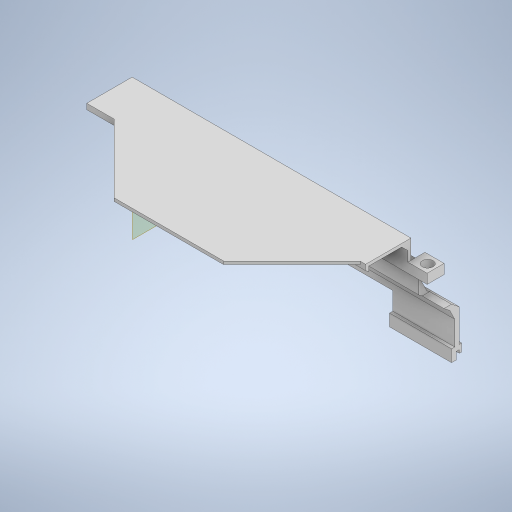
# Autodesk Inventor part: kryt
Saved by Autodesk Inventor 2024 (Build 280153000, 153)
## iProperties
Created: 2023-09-06
Part Number: kryt
Material: Všeobecné
Document SubType Name: Modeling
Designer: Simak
Density: 1 g/cm^3
Appearance: Výchozí
Author: Simak
Autodesk Inventor part; units mm, degrees
ref_plane "YZ Plane" through (0, 0, 0) normal (1, 0, 0) x (0, 1, 0)
ref_plane "XZ Plane" through (0, 0, 0) normal (0, 1, 0) x (-1, 0, 0)
ref_plane "XY Plane" through (0, 0, 0) normal (0, 0, 1) x (1, 0, 0)
ref_plane "Pracovní rovina12" through (0, 3, 0) normal (0, 1, 0) x (1, 0, 0)
sketch "Náčrt28" plane through (0, 3, 0) normal (0, 1, 0) x (1, 0, 0)
  circle A0 centre (-42.25, 8.5) radius 1.85
  circle A1 centre (42.25, 8.5) radius 1.85
  circle A2 centre (42.25, -29) radius 1.85
  circle A3 centre (-42.25, -29) radius 1.85
  line L0 (-42.25, 8.5) -> (-49.75, 8.5) construction
  line L1 (-49.75, 19.25) -> (-49.75, -49.75) projected
  line L2 (42.25, 8.5) -> (49.75, 8.5) construction
  line L3 (49.75, -49.75) -> (49.75, 19.25) projected
  line L4 (-49.75, -49.75) -> (49.75, -49.75) projected
  point P0 (0, 0)
  dimension "d185" = 3.7
  dimension "d186" = 84.5
  dimension "d187" = 37.5
  dimension "d195" = 20.75
  constraints: 4 centre point, 4 end point, 3 equal radius, 3 point on line, 2 horizontal alignment, 2 vertical alignment, 1 collinear, 1 horizontal
  measures "d185" diameter of A0
  measures "d186" distance of L2.start L0.start
  measures "d187" distance of A3.centre L0.start
  measures "d195" distance from line of L4 A3.centre
ref_plane "Pracovní rovina6" through (49.75, 0, 49.75) normal (1, 0, 0) x (0, 0, -1)
sketch "Náčrt29" plane through (49.75, 0, 49.75) normal (1, 0, 0) x (0, 0, -1)
  line L0 (0, 0) -> (69, 0) projected
  line L1 (0, 0) -> (6.6987, 25)
  line L2 (6.6987, 25) -> (9.8046, 25)
  line L3 (9.8046, 25) -> (3.9097, 3)
  line L4 (0, 3) -> (69, 3) projected
  line L5 (0, 0) -> (0, 3) projected
  point P0 (49.75, 0)
  point P1 (0.8038, 3)
  dimension "d188" = 75
  dimension "d189" = 25
  dimension "d190" = 3
  constraints: 6 end point, 1 horizontal, 1 parallel, 1 point on line
  measures "d188" angle of L0 L1
  measures "d189" distance between parallel lines of L0 L2
  measures "d190" distance between parallel lines of L1 L3
ref_plane "Pracovní rovina7" through (-49.75, 25, 5) normal (0, 0, 1) x (1, 0, 0)
sketch "Náčrt49" plane through (-49.75, 25, 5) normal (0, 0, 1) x (1, 0, 0)
  line L0 (0, 0) -> (2.5, 0) projected
  line L1 (1.25, 0) -> (4.45, 0)
  line L2 (4.45, 0) -> (4.45, 5.2)
  line L3 (4.45, 5.2) -> (1.25, 5.2)
  line L4 (1.25, 5.2) -> (1.25, 0)
  line L5 (2.5, 7.2) -> (6.45, 7.2)
  line L6 (6.45, 7.2) -> (6.45, -2)
  line L7 (6.45, -2) -> (2.5, -2)
  line L8 (2.5, 7.2) -> (2.5, 5.2)
  line L9 (2.5, 0) -> (2.5, -12) projected
  line L10 (2.5, 0) -> (2.5, -2)
  line L11 (2.5, 0) -> (2.5, 19) projected
  point P0 (49.75, -25)
  point P1 (1.25, 0)
  point P2 (2.5, 0)
  point P3 (2.5, 0)
  dimension "d289" = 3.2
  dimension "d290" = 5.2
  dimension "d291" = 2
  dimension "d292" = 2
  dimension "d293" = 2
  constraints: 18 end point, 3 perpendicular, 2 collinear, 2 horizontal, 2 midpoint, 2 parallel, 1 point on line, 1 vertical, 1 vertical alignment
  measures "d289" distance of L2.end L3.end
  measures "d290" distance of L1.end L2.end
  measures "d291" distance between parallel lines of L1 L7
  measures "d292" distance between parallel lines of L6 L2
  measures "d293" distance between parallel lines of L3 L5
ref_plane "Pracovní rovina14" through (0, 0, 0) normal (0, -1, 0) x (1, 0, 0)
sketch "Náčrt53" plane through (0, 0, 0) normal (0, -1, 0) x (1, 0, 0)
  line L0 (5, -49.75) -> (-5, -49.75) projected
  line L1 (-5, -49.75) -> (-5, -39.875) projected
  line L2 (-5, -39.875) -> (5, -39.875) projected
  line L3 (5, -39.875) -> (5, -49.75) projected
  line L4 (0, -48.0745) -> (-2.825, -46.4435)
  line L5 (-2.825, -46.4435) -> (-2.825, -43.1815)
  line L6 (-2.825, -43.1815) -> (0, -41.5505)
  line L7 (0, -41.5505) -> (2.825, -43.1815)
  line L8 (2.825, -43.1815) -> (2.825, -46.4435)
  line L9 (2.825, -46.4435) -> (0, -48.0745)
  line L10 (0, -48.0745) -> (0, -49.75) construction
  line L11 (0, -41.5505) -> (0, -39.875) construction
  circle A0 centre (0, -44.8125) radius 1.85
  point P0 (0, 0)
  point P1 (0, -44.8125)
  dimension "d328" = 3.7
  dimension "d389" = 5.65
  constraints: 16 end point, 2 midpoint, 1 centre point, 1 coincident, 1 collinear, 1 vertical, 1 vertical alignment, 13 other
  measures "d328" diameter of A0
  measures "d389" distance between parallel lines of L8 L5
ref_plane "Pracovní rovina10" through (27, 7.646, -39.875) normal (1, 0, 0) x (0, 0, -1)
sketch "Náčrt72" plane through (27, 7.646, -39.875) normal (1, 0, 0) x (0, 0, -1)
  line L0 (-1.9585, -1.746) -> (-8.7915, -1.746)
  line L1 (-8.7915, 8.454) -> (-1.9585, 8.454)
  arc A0 (-8.7915, 8.454) -> (-8.7915, -1.746) centre (-5.375, 3.354) ccw
  arc A1 (-1.9585, -1.746) -> (-1.9585, 8.454) centre (-5.375, 3.354) ccw
  line L2 (-9, -7.646) -> (-1, -7.646) projected
  line L3 (-10.75, 0) -> (-10.75, 3.354) projected
  arc A2 (-10.75, 0) -> (-5.375, -3.1882) centre (-5.375, 2.9368) ccw projected
  arc A3 (-5.375, -3.1882) -> (0, 0) centre (-5.375, 2.9368) ccw projected
  line L4 (0, 3.354) -> (0, 0) projected
  line L5 (-10.75, 3.354) -> (0, 3.354)
  line L6 (-13.75, -3.1882) -> (-5.375, -3.1882) projected
  line L7 (-13.75, -3.1882) -> (-13.75, -1.746)
  line L8 (-13.8375, 3.354) -> (-13.8375, -7.646) projected
  line L9 (-13.75, -1.746) -> (-8.7915, -1.746)
  point P0 (-39.875, -7.646)
  point P1 (-5.375, -1.746)
  point P2 (-9.7183, -1.3819)
  point P3 (-11.5136, 3.354)
  point P4 (-10.75, 0.3889)
  point P5 (0, 0.3889)
  point P6 (-9.323, -1.746)
  point P7 (-5.375, 8.454)
  dimension "d190" = 3
  dimension "d447" = 6.833
  dimension "d448" = 10.2
  constraints: 10 end point, 5 point on circle, 3 midpoint, 2 centre point, 2 coincident, 2 parallel, 2 vertical alignment, 1 collinear
  measures "d447" distance of L1.start L1.end
  measures "d448" distance between parallel lines of L0 L1
ref_plane "Pracovní rovina11" through (0, 3, 0) normal (0, 1, 0) x (1, 0, 0)
sketch "Náčrt74" plane through (0, 3, 0) normal (0, 1, 0) x (1, 0, 0)
  line L0 (-17, 18.25) -> (17, 18.25)
  line L1 (-17, 26.125) -> (-17, 18.25) projected
  line L2 (-12, 26.125) -> (-17, 26.125) projected
  line L3 (-12, 26.125) -> (-12, 39.875) projected
  line L4 (12, 39.875) -> (-12, 39.875) projected
  line L5 (12, 26.125) -> (12, 39.875) projected
  line L6 (17, 26.125) -> (12, 26.125) projected
  line L7 (17, 18.25) -> (17, 26.125) projected
  line L8 (-5, 49.75) -> (-5, 39.875) projected
  line L9 (5, 39.875) -> (5, 49.75) projected
  line L10 (-5, 39.875) -> (-5, 35.875)
  arc A0 (-5, 35.875) -> (5, 35.875) centre (0, 35.875) ccw
  line L11 (5, 35.875) -> (5, 39.875)
  line L12 (-12, 35.875) -> (-5, 35.875)
  line L13 (5, 35.875) -> (12, 35.875)
  line L14 (-27, 39.75) -> (27, 39.75) projected
  line L15 (-8, 39.875) -> (-8, 33.875)
  line L16 (-8, 33.875) -> (-17, 33.875)
  line L17 (-17, 29.125) -> (-17, 34.5) projected
  line L18 (8, 39.875) -> (8, 33.875)
  line L19 (8, 33.875) -> (17, 33.875)
  line L20 (-17, 19.25) -> (-17, 29.125) projected
  line L21 (17, 29.125) -> (17, 19.25) projected
  line L22 (17, 34.5) -> (17, 29.125) projected
  line L23 (-8, 33.875) -> (-8, 26.125)
  line L24 (-8, 26.125) -> (-12, 26.125)
  line L25 (8, 33.875) -> (8, 26.125)
  line L26 (8, 26.125) -> (12, 26.125)
  point P0 (0, 0)
  point P1 (0, 30.875)
  point P2 (5, 35.875)
  point P3 (-5, 35.875)
  point P4 (12, 33.875)
  point P5 (8, 39.75)
  point P6 (12, 39.75)
  point P7 (-12, 39.75)
  point P8 (-8, 39.75)
  point P9 (-12, 33.875)
  point P10 (8, 35.875)
  point P11 (-8, 35.875)
  point P12 (5, 39.75)
  point P13 (-5, 39.75)
  dimension "d458" = 5
  dimension "d464" = 8.875
  dimension "d465" = 3
  dimension "d466" = 3
  dimension "d467" = 6
  constraints: 26 end point, 8 point on line, 6 perpendicular, 5 point on circle, 4 vertical, 2 equal length, 1 centre point, 1 coincident, 1 horizontal, 1 tangent
  measures "d458" radius of A0
  measures "d464" distance from line of point (0, 30.875) L14
  measures "d465" distance between parallel lines of L10 L15
  measures "d466" distance between parallel lines of L18 L11
  measures "d467" distance between parallel lines of L4 L19
ref_plane "Pracovní rovina8" through (47.25, 44, 5) normal (0, 1, 0) x (1, 0, 0)
sketch "Náčrt63" plane through (47.25, 44, 5) normal (0, 1, 0) x (1, 0, 0)
  line L0 (0, 20.75) -> (0, 10) projected
  line L1 (0, 14.65) -> (-6.75, 14.65)
  line L2 (2.5, 2) -> (-6.75, 2) projected
  line L3 (-6.75, 2) -> (-6.75, 0) projected
  line L4 (2.5, 2) -> (2.5, 24.25) projected
  line L5 (2.5, 18.15) -> (-6.75, 18.15)
  line L6 (-6.75, 18.15) -> (-6.75, 14.65)
  line L7 (0, 2) -> (0, 24.25) projected
  point P0 (-47.25, 5)
  point P1 (0, 18.15)
  dimension "d190" = 3
  dimension "d408" = 12.65
  dimension "d413" = 3.5
  constraints: 6 end point, 2 horizontal, 2 point on line, 1 perpendicular, 1 vertical alignment
  measures "d408" distance between parallel lines of L1 L2
  measures "d413" distance of L5.end L1.end
ref_plane "Pracovní rovina9" through (47.25, 44, 5) normal (0, 1, 0) x (1, 0, 0)
sketch "Náčrt64" plane through (47.25, 44, 5) normal (0, 1, 0) x (1, 0, 0)
  circle A0 centre (-3.375, 17.4) radius 1.75
  line L0 (-6.75, 14.65) -> (0, 14.65) projected
  line L1 (0, 14.65) -> (-3.375, 17.4) construction
  line L2 (-3.375, 17.4) -> (-6.75, 14.65) construction
  line L3 (-5.125, 17.4) -> (-5.125, 18.15)
  line L4 (2.5, 18.15) -> (-6.75, 18.15) projected
  line L5 (-1.625, 17.4) -> (-1.625, 18.15)
  point P0 (-47.25, 5)
  dimension "d414" = 3.5
  dimension "d415" = 2.75
  constraints: 8 end point, 2 point on circle, 2 point on line, 2 tangent, 1 centre point, 1 equal length, 1 perpendicular, 1 vertical
  measures "d414" diameter of A0
  measures "d415" distance from line of L0 L1.end
ref_plane "Pracovní rovina5" through (45.625, 37.275, -13.15) normal (0, 1, 0) x (1, 0, 0)
sketch "Náčrt67" plane through (45.625, 37.275, -13.15) normal (0, 1, 0) x (1, 0, 0)
  arc A0 (-3.5, -0.75) -> (0, -0.75) centre (-1.75, -0.75) ccw projected
  line L0 (-4.7811, -0.75) -> (-3.2655, 1.875)
  line L1 (-3.2655, 1.875) -> (-0.2345, 1.875)
  line L2 (-0.2345, 1.875) -> (1.2811, -0.75)
  line L3 (1.2811, -0.75) -> (-0.2345, -3.375)
  line L4 (-0.2345, -3.375) -> (-3.2655, -3.375)
  line L5 (-3.2655, -3.375) -> (-4.7811, -0.75)
  circle A1 centre (-1.75, -0.75) radius 1.75
  point P0 (-45.625, -13.15)
  dimension "d423" = 5.25
  constraints: 12 end point, 2 coincident, 1 horizontal alignment, 16 other
  measures "d423" distance between parallel lines of L4 L1
ref_plane "Pracovní rovina13" through (40.5, 44, -9.65) normal (0, 0, 1) x (1, 0, 0)
sketch "Náčrt71" plane through (40.5, 44, -9.65) normal (0, 0, 1) x (1, 0, 0)
  line L0 (3.625, -5.225) -> (4.8905, -6.4905) projected
  line L1 (3.625, -5.225) -> (4.8905, -5.225) projected
  line L2 (4.8905, -6.4905) -> (4.8905, -5.225) projected
  line L3 (0, -1.6) -> (6.75, -8.35) projected
  line L4 (1.8595, -5.225) -> (3.625, -5.225) projected
  line L5 (1.8595, -3.4595) -> (3.625, -5.225) projected
  line L6 (1.8595, -5.225) -> (1.8595, -3.4595) projected
  point P0 (-40.5, -44)
ref_plane "Pracovní rovina15" through (-47.25, 13, -19.25) normal (1, 0, 0) x (0, 0, -1)
sketch "Náčrt80" plane through (-47.25, 13, -19.25) normal (1, 0, 0) x (0, 0, -1)
  line L0 (-63.2878, -3.273) -> (-63.8446, -3.8298) projected
  line L1 (-63.8446, -5.351) -> (-63.8446, -3.8298) projected
  line L2 (-64.5544, -8) -> (-63.8446, -5.351) projected
  line L3 (-64.5544, -8) -> (-53.75, -8) projected
  line L4 (-53.75, -5.5) -> (-53.75, -8) projected
  line L5 (-53.75, -5.5) -> (-45.0078, -5.5) projected
  arc A0 (-42.098, 1.44) -> (-45.0078, -5.5) centre (-42.098, -2.64) ccw projected
  line L6 (-42.098, 1.44) -> (-36.318, 1.44) projected
  arc A1 (-36.318, -6.72) -> (-36.318, 1.44) centre (-36.318, -2.64) ccw projected
  line L7 (-36.318, -6.72) -> (-42.098, -6.72) projected
  arc A2 (-42.75, -6.6676) -> (-42.098, -6.72) centre (-42.098, -2.64) ccw projected
  line L8 (-42.75, -8) -> (-42.75, -6.6676) projected
  line L9 (-42.75, -8) -> (-16.25, -8) projected
  line L10 (-16.25, -5.5) -> (-16.25, -8) projected
  line L11 (-16.25, -5.5) -> (-3.5, -5.5) projected
  line L12 (-3.5, -5.5) -> (-1, -3) projected
  line L13 (-1, -3) -> (-1, 0) projected
  line L14 (-1, 0) -> (0, 0) projected
  line L15 (0, 12) -> (0, 0) projected
  line L16 (-24.25, 31) -> (0, 12) projected
  line L17 (-24.25, 19.2) -> (-24.25, 31) projected
  line L18 (-24.25, 19.2) -> (-12.05, 19.2) projected
  line L19 (-12.05, 19.2) -> (-12.05, 6.05) projected
  line L20 (-24.25, 6.05) -> (-12.05, 6.05) projected
  line L21 (-24.25, 6.05) -> (-24.25, 12) projected
  line L22 (-24.25, 12) -> (-59.1954, 12) projected
  line L23 (-63.2878, -3.273) -> (-59.1954, 12) projected
  line L24 (0, -8) -> (0, 12) projected
  line L25 (-1.5, 11.2697) -> (-1.5, 1.5)
  line L26 (-1.5, 1.5) -> (-2.5, 1.5)
  line L27 (-2.5, 1.5) -> (-2.5, -2.3787)
  line L28 (-2.5, -2.3787) -> (-4.1213, -4)
  line L29 (-4.1213, -4) -> (-17.75, -4)
  line L30 (-17.75, -4) -> (-17.75, -6.5)
  line L31 (-17.75, -6.5) -> (-41.25, -6.5)
  line L32 (-41.25, -6.5) -> (-41.25, -8.1552)
  arc A3 (-41.25, -8.1552) -> (-42.098, -8.22) centre (-42.098, -2.64) ccw
  line L33 (-42.098, -8.22) -> (-36.318, -8.22)
  arc A4 (-36.318, -8.22) -> (-36.318, 2.94) centre (-36.318, -2.64) ccw
  line L34 (-36.318, 2.94) -> (-42.098, 2.94)
  arc A5 (-42.098, 2.94) -> (-47.5097, -4) centre (-42.098, -2.64) ccw
  line L35 (-47.5097, -4) -> (-55.25, -4)
  line L36 (-55.25, -4) -> (-55.25, -6.5)
  line L37 (-55.25, -6.5) -> (-62.5996, -6.5)
  line L38 (-62.5996, -6.5) -> (-62.3446, -5.5485)
  line L39 (-62.3446, -5.5485) -> (-62.3446, -4.4511)
  line L40 (-62.3446, -4.4511) -> (-61.943, -4.0495)
  line L41 (-61.943, -4.0495) -> (-58.0445, 10.5)
  line L42 (-58.0445, 10.5) -> (-25.75, 10.5)
  line L43 (-25.75, 10.5) -> (-25.75, 4.55)
  line L44 (-25.75, 4.55) -> (-10.55, 4.55)
  line L45 (-10.55, 4.55) -> (-10.55, 18.3604)
  line L46 (-22.75, 20.7) -> (-22.75, 27.9192)
  line L47 (-22.75, 27.9192) -> (-1.5, 11.2697)
  line L48 (-13.5361, 20.7) -> (-22.75, 20.7)
  line L49 (-2.5, -2.3787) -> (0.75, -2.3787)
  line L50 (0.75, -2.3787) -> (0.75, 1.5)
  line L51 (0.75, 1.5) -> (-1.5, 1.5)
  line L52 (-22.75, 27.9192) -> (-24.25, 29.0944)
  line L53 (-63.8446, -3.8298) -> (-63.2878, -3.273) projected
  line L54 (-59.1954, 12) -> (-63.2878, -3.273) projected
  line L55 (-24.25, 12) -> (-59.1954, 12) projected
  line L56 (-24.25, 12) -> (-24.25, 6.05) projected
  line L57 (-12.05, 6.05) -> (-24.25, 6.05) projected
  line L58 (-12.05, 6.05) -> (-12.05, 19.2) projected
  line L59 (-24.25, 19.2) -> (-12.05, 19.2) projected
  line L60 (-24.25, 19.2) -> (-24.25, 22.65) projected
  line L61 (-24.25, 22.65) -> (-22.25, 22.65) projected
  line L62 (-22.25, 31) -> (-22.25, 22.65) projected
  line L63 (-9.6, 31) -> (-22.25, 31) projected
  line L64 (-9.6, 31) -> (-9.6, 22.65) projected
  line L65 (-9.6, 22.65) -> (-6.1, 22.65) projected
  line L66 (-6.1, 22.65) -> (-6.1, 17) projected
  line L67 (-6.3816, 17) -> (-6.1, 17) projected
  line L68 (-6.3816, 17) -> (0, 12) projected
  line L69 (0, 0) -> (0, 12) projected
  line L70 (0, 0) -> (-1, 0) projected
  line L71 (-1, 0) -> (-1, -3) projected
  line L72 (-1, -3) -> (-3.5, -5.5) projected
  line L73 (-3.5, -5.5) -> (-16.25, -5.5) projected
  line L74 (-16.25, -8) -> (-16.25, -5.5) projected
  line L75 (-16.25, -8) -> (-42.75, -8) projected
  line L76 (-42.75, -5.5) -> (-42.75, -8) projected
  line L77 (-42.75, -5.5) -> (-53.75, -5.5) projected
  line L78 (-53.75, -8) -> (-53.75, -5.5) projected
  line L79 (-53.75, -8) -> (-64.5544, -8) projected
  line L80 (-63.8446, -5.351) -> (-64.5544, -8) projected
  line L81 (-63.8446, -5.351) -> (-63.8446, -3.8298) projected
  line L82 (-8.6, 23.65) -> (-8.6, 32)
  line L83 (-8.6, 32) -> (-23.25, 32)
  line L84 (-23.25, 32) -> (-23.25, 23.65)
  line L85 (-23.25, 23.65) -> (-25.25, 23.65)
  line L86 (-25.25, 23.65) -> (-25.25, 18.2)
  line L87 (-25.25, 18.2) -> (-13.05, 18.2)
  line L88 (-13.05, 18.2) -> (-13.05, 7.05)
  line L89 (-13.05, 7.05) -> (-23.25, 7.05)
  line L90 (-23.25, 7.05) -> (-23.25, 13)
  line L91 (-23.25, 13) -> (-59.9628, 13)
  line L92 (-59.9628, 13) -> (-64.1844, -2.7554)
  line L93 (-64.1844, -2.7554) -> (-64.8446, -3.4156)
  line L94 (-64.8446, -3.4156) -> (-64.8446, -5.2194)
  line L95 (-64.8446, -5.2194) -> (-65.8577, -9)
  line L96 (-65.8577, -9) -> (-52.75, -9)
  line L97 (-52.75, -9) -> (-52.75, -6.5)
  line L98 (-52.75, -6.5) -> (-43.75, -6.5)
  line L99 (-43.75, -6.5) -> (-43.75, -9)
  line L100 (-43.75, -9) -> (-15.25, -9)
  line L101 (-15.25, -9) -> (-15.25, -6.5)
  line L102 (-15.25, -6.5) -> (-3.0858, -6.5)
  line L103 (-3.0858, -6.5) -> (0, -3.4142)
  line L104 (0, -3.4142) -> (0, -1)
  line L105 (0, -1) -> (1, -1)
  line L106 (1, -1) -> (1, 12.4869)
  line L107 (1, 12.4869) -> (-5.1, 17.2663)
  line L108 (-5.1, 17.2663) -> (-5.1, 23.65)
  line L109 (-5.1, 23.65) -> (-8.6, 23.65)
  line L110 (-6.1, 17) -> (-6.1, 14.8738)
  line L111 (-5.1, 17.2663) -> (-5.1, 14.0903)
  point P0 (-19.25, -13)
  point P1 (-1, -2.3787)
  point P2 (0, -1)
  point P3 (0.75, -1)
  point P4 (0, 1.5)
  point P5 (-5.1, 15.9959)
  point P6 (-23.25, 30.2165)
  point P7 (-22.25, 29.433)
  dimension "d491" = 1.5
  dimension "d492" = 5.58
  dimension "d493" = 10.55
  dimension "d494" = 20.7
  dimension "d495" = 0.75
  dimension "d496" = 1
  constraints: 116 end point, 6 point on circle, 5 point on line, 3 centre point, 2 parallel, 2 perpendicular, 2 vertical, 1 collinear, 1 horizontal, 50 other
  measures "d491" distance between parallel lines of L47 L16
  measures "d492" radius of A4
  measures "d493" distance between parallel lines of L15 L45
  measures "d494" distance between parallel lines of L14 L48
  measures "d495" distance between parallel lines of L24 L50
  measures "d496" distance between parallel lines of L64 L82
extrude "Vysunutí84" add sketch "Náčrt80" along normal blind 94.5 contours L84 L83 L82 L109 L108 L111 L16 L110 L66 L65 L64 L63 L62 | L110 L16 L111 L47 | L111 L16 L15 L51 L25 L47 | L27 L26 L51 L15 L14 L13 L49 | L24 L15 L51 L50 L105
ref_plane "Pracovní rovina16" through (-47.25, 13, -19.25) normal (-1, 0, 0) x (0, 0, 1)
sketch "Náčrt81" plane through (-47.25, 13, -19.25) normal (-1, 0, 0) x (0, 0, 1)
  line L0 (6.1, 22.65) -> (6.1, 14.8738) projected
  line L1 (9.6, 22.65) -> (6.1, 22.65) projected
  line L2 (9.6, 31) -> (9.6, 22.65) projected
  line L3 (22.25, 31) -> (9.6, 31) projected
  line L4 (22.25, 29.433) -> (22.25, 31) projected
  line L5 (23.25, 30.2165) -> (22.25, 29.433) projected
  line L6 (23.25, 32) -> (23.25, 30.2165) projected
  line L7 (8.6, 32) -> (23.25, 32) projected
  line L8 (8.6, 23.65) -> (8.6, 32) projected
  line L9 (5.1, 23.65) -> (8.6, 23.65) projected
  line L10 (5.1, 15.9959) -> (5.1, 23.65) projected
  line L11 (0, -8) -> (67.6603, -8) projected
  line L12 (67.6603, -8) -> (62.3013, 12) projected
  line L13 (24.25, 12) -> (62.3013, 12) projected
  line L14 (24.25, 12) -> (24.25, 31) projected
  line L15 (24.25, 31) -> (0, 12) projected
  line L16 (0, -8) -> (0, 12) projected
  arc A0 (42.098, -6.72) -> (42.098, 1.44) centre (42.098, -2.64) ccw projected
  line L17 (42.098, -6.72) -> (36.318, -6.72) projected
  arc A1 (36.318, 1.44) -> (36.318, -6.72) centre (36.318, -2.64) ccw projected
  line L18 (36.318, 1.44) -> (42.098, 1.44) projected
  line L19 (2.5, -2.3787) -> (1, -2.3787) projected
  line L20 (2.5, 1.5) -> (2.5, -2.3787) projected
  line L21 (1.5, 1.5) -> (2.5, 1.5) projected
  line L22 (1.5, 11.2697) -> (1.5, 1.5) projected
  line L23 (6.1, 14.8738) -> (1.5, 11.2697) projected
  line L24 (0, 12) -> (5.1, 15.9959) projected
  line L25 (0, 1.5) -> (0, 12) projected
  line L26 (-0.75, 1.5) -> (0, 1.5) projected
  line L27 (-0.75, -1) -> (-0.75, 1.5) projected
  line L28 (0, -1) -> (-0.75, -1) projected
  line L29 (0, 0) -> (0, -1) projected
  line L30 (1, 0) -> (0, 0) projected
  line L31 (1, -2.3787) -> (1, 0) projected
  point P0 (19.25, -13)
  point P1 (5.1, 15.9959)
  point P2 (6.1, 16.7794)
extrude "Vysunutí85" add sketch "Náčrt81" along normal blind 2.5 contours L1 L2 L3 L4 L15 L0 | L0 L15 L10 L9 L8 L7 L6 L5 L4 L3 L2 L1
sketch "Náčrt82" plane through (-47.25, 12, -20) normal (0, 0, -1) x (-1, 0, 0)
  line L0 (-74.5, -5.1099) -> (-20, -5.1099)
  line L1 (-20, -5.1099) -> (-20, 8.3236)
  line L2 (-20, 8.3236) -> (-74.5, 8.3236)
  line L3 (-74.5, 8.3236) -> (-74.5, -5.1099)
  line L4 (0, 42) -> (0, -21) projected
  line L5 (-94.5, 2.5) -> (-94.5, 13) projected
  point P0 (-47.25, -12)
  dimension "d501" = 20
  dimension "d502" = 20
  dimension "d503" = 13.4335
  dimension "d504" = 33.6764
  constraints: 8 end point, 2 parallel, 1 horizontal, 1 perpendicular
  measures "d501" distance between parallel lines of L4 L1
  measures "d502" distance between parallel lines of L5 L3
  measures "d503" distance between parallel lines of L2 L0
  measures "d504" distance from line of L4.start L2
extrude "Vysunutí86" cut sketch "Náčrt82" against normal blind 94.5
sketch "Náčrt83" plane through (47.25, 28.9959, -14.15) normal (0, 0, -1) x (-1, 0, 0)
  line L0 (97, 16.0041) -> (0, 16.0041) projected
  line L1 (0, 16.0041) -> (7, 16.0041)
  line L2 (7, 16.0041) -> (7, -1.9959)
  line L3 (7, -1.9959) -> (0, -1.9959)
  line L4 (0, -1.9959) -> (0, 16.0041)
  point P0 (47.25, -28.9959)
  point P1 (0, -1.9959)
  dimension "d507" = 7
  dimension "d537" = 18
  constraints: 8 end point, 2 parallel, 1 horizontal, 1 perpendicular, 1 point on line
  measures "d507" distance between parallel lines of L4 L2
  measures "d537" distance of L3.end L0.end
extrude "Vysunutí87" cut sketch "Náčrt83" along normal through all both and the other way through all
sketch "Náčrt84" plane through (-49.75, 45, 4) normal (0, 1, 0) x (1, 0, 0)
  line L0 (66.197, -22) -> (30.803, -22)
  line L1 (30.803, -22) -> (8.803, 0)
  line L2 (66.197, -22) -> (88.197, 0)
  line L3 (8.803, 0) -> (0, 0)
  line L4 (97, 0) -> (88.197, 0)
  line L5 (0, 0) -> (90, 0) projected
  line L6 (97, 20.6974) -> (97, 18.2652) projected
  point P0 (49.75, 4)
  point P1 (97, 17.65)
  point P2 (97, 18.15)
  point P3 (97, 17.15)
  dimension "d513" = 22
  dimension "d514" = 45
  dimension "d515" = 45
  dimension "d516" = 90
  dimension "d517" = 6.6093
  constraints: 10 end point, 2 horizontal, 2 point on line, 1 collinear, 1 vertical alignment
  measures "d513" distance between parallel lines of L5 L0
  measures "d514" angle of L5 L1
  measures "d515" angle of L5 L2
  measures "d516" angle of L3 L6
  measures "d517" distance from line of point (97, 18.15) L2
extrude "Vysunutí88" add sketch "Náčrt84" against normal up to surface (1 mm away)
sketch "Náčrt85" plane through (40.25, 28.9959, -14.15) normal (1, 0, 0) x (0, 0, -1)
  line L0 (-4.5, 6.6541) -> (1, 6.6541)
  line L1 (1, 6.6541) -> (1, 9.7791)
  line L2 (1, 9.7791) -> (-4.5, 9.7791)
  line L3 (-4.5, 9.7791) -> (-4.5, 6.6541)
  line L4 (0, 7.6541) -> (0, 0) projected
  line L5 (-3.5, 7.6541) -> (0, 7.6541) projected
  point P0 (-14.15, -28.9959)
  point P1 (-1, 6.6541)
  point P2 (-4.5, 6.6541)
  dimension "d520" = 1
  dimension "d521" = 2.125
  constraints: 8 end point, 2 parallel, 2 point on line, 1 horizontal, 1 perpendicular
  measures "d520" distance between parallel lines of L4 L1
  measures "d521" distance between parallel lines of L2 L5
extrude "Vysunutí89" add sketch "Náčrt85" along normal blind 6.2
sketch "Náčrt86" plane through (40.25, 38.775, -10.65) normal (0, 1, 0) x (1, 0, 0)
  line L0 (0, 4.5) -> (6.2, 4.5) projected
  line L1 (0, 4.5) -> (0, 0) projected
  point P0 (-40.25, -10.65)
  point P1 (3.65, 1.75)
  dimension "d525" = 2.75
  dimension "d526" = 3.65
  measures "d525" distance from line of L0 point (3.65, 1.75)
  measures "d526" distance from line of L1 point (3.65, 1.75)
hole "Díra4" at (43.9, 38.775, -12.4) direction (0, -1, 0) diameter 3.5 end up to face face through (13.15, 35.65, -10.8167) facing (0, -1, 0)
chamfer "Zkosení18" distance 2 angle 45 6 edges at (40.25, 36.65, -12.4) (-4.75, 36.65, -10.65) (-3.5, 28.9959, -14.15) (0, 24.2697, -17.75) (-3.5, 35.65, -13.15) (-3.5, 44, -9.65)
